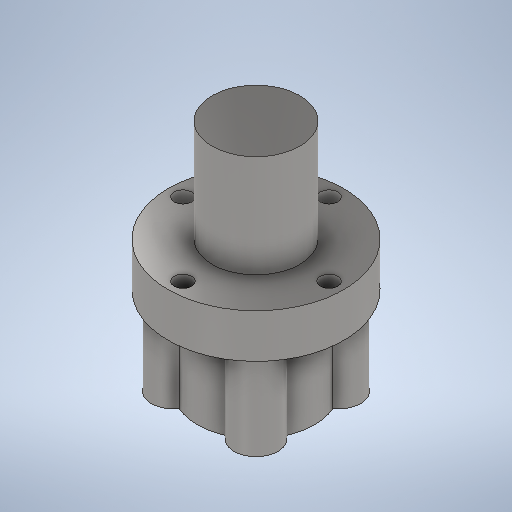
# Autodesk Inventor part: Крепление Барабана2
Saved by Autodesk Inventor 2025.1 (Build 291241000, 241)
## iProperties
Created: 2025-03-01
Part Number: Крепление Барабана2
Material: Сталь, литейная
Document SubType Name: Modeling
Designer: Timofey
Density: 7.85 g/cm^3
Appearance: С умеренной полировкой
Mass: 2001.3 g
Surface Area: 306.52 cm^2
Volume: 254.942 cm^3
Author: Timofey
Autodesk Inventor part; units mm, degrees
ref_plane "YZ Plane" through (0, 0, 0) normal (1, 0, 0) x (0, 1, 0)
ref_plane "XZ Plane" through (0, 0, 0) normal (0, 1, 0) x (-1, 0, 0)
ref_plane "XY Plane" through (0, 0, 0) normal (0, 0, 1) x (1, 0, 0)
sketch "Эскиз1" plane through (0, 0, 0) normal (0, 1, 0) x (-1, 0, 0)
  circle A0 centre (0, 0) radius 30
  dimension "d0" = 60
  constraints: 1 centre point, 1 coincident
  measures "d0" diameter of A0
extrude "Выдавливание1" add sketch "Эскиз1" along normal blind 15
sketch "Эскиз3" plane through (0, 0, 0) normal (0, -1, 0) x (1, 0, 0)
  circle A0 centre (0, 0) radius 20
  line L0 (0, 0) -> (30, 0) construction
  line L1 (0, 0) -> (30, 0) construction
  line L2 (0, 0) -> (30, 0) construction
  line L3 (0, 0) -> (30, 0) construction
  line L4 (0, 0) -> (14.1421, 14.1421)
  line L5 (0, 0) -> (20, 0) construction
  line L6 (0, 0) -> (14.1421, -14.1421)
  line L7 (0, 0) -> (-14.1421, 14.1421)
  line L8 (0, 0) -> (20, 0) construction
  line L9 (0, 0) -> (-14.1421, -14.1421)
  line L10 (0, 0) -> (20, 0) construction
  circle A1 centre (14.1421, 14.1421) radius 7.5
  circle A2 centre (14.1421, -14.1421) radius 7.5
  circle A3 centre (-14.1421, -14.1421) radius 7.5
  circle A4 centre (-14.1421, 14.1421) radius 7.5
  point P0 (-8.7707, -17.9743)
  point P1 (-16.2945, -11.5969)
  point P2 (-8.7707, 17.9743)
  point P3 (-16.2945, 11.5969)
  point P4 (11.5969, -16.2945)
  point P5 (17.9743, -8.7707)
  point P6 (17.995, 8.7282)
  point P7 (11.5862, 16.3021)
  point P8 (18.357, 7.9385)
  point P9 (7.9385, 18.357)
  point P10 (-7.9385, 18.357)
  point P11 (-18.357, 7.9385)
  point P12 (-18.357, -7.9385)
  point P13 (-7.9385, -18.357)
  point P14 (7.9385, -18.357)
  point P15 (18.357, -7.9385)
  dimension "d26" = 40
  dimension "d62" = 20
  dimension "d63" = 45
  dimension "d64" = 20
  dimension "d65" = 20
  dimension "d66" = 135
  dimension "d67" = 20
  dimension "d68" = 135
  dimension "d69" = 15
  dimension "d70" = 15
  dimension "d71" = 15
  dimension "d72" = 15
  constraints: 22 end point, 7 horizontal, 4 centre point, 3 coincident, 3 equal length, 2 point on line, 1 collinear, 1 perpendicular, 12 other
  measures "d62" distance of L0.start L4.end
  measures "d63" angle of L5 L4
  measures "d64" distance of L0.start L6.end
  measures "d65" distance of L0.start L7.end
  measures "d66" angle of L8 L7
  measures "d67" distance of L0.start L9.end
  measures "d68" angle of L9 L10
  measures "d69" diameter of A1
  measures "d70" diameter of A2
  measures "d71" diameter of A3
  measures "d72" diameter of A4
sketch "Эскиз4" plane through (0, 15, 0) normal (0, 1, 0) x (1, 0, 0)
  circle A0 centre (0, 0) radius 15
  dimension "d41" = 30
  constraints: 1 centre point, 1 coincident
  measures "d41" diameter of A0
extrude "Выдавливание3" add sketch "Эскиз4" along normal blind 35
sketch "Эскиз5" plane through (0, 15, 0) normal (0, 1, 0) x (1, 0, 0)
  line L0 (0, 0) -> (0, -25)
  arc A0 (20, 0) -> (20, 0) centre (0, 0) ccw projected
  line L1 (0, 0) -> (25, 0)
  line L2 (0, 0) -> (0, 25)
  line L3 (0, 0) -> (-25, 0)
  dimension "d44" = 25
  dimension "d45" = 25
  dimension "d46" = 25
  dimension "d47" = 25
  constraints: 8 end point, 2 horizontal, 2 vertical
  measures "d44" distance of L0.start L0.end
  measures "d45" distance of L1.start L1.end
  measures "d46" distance of L1.start L2.end
  measures "d47" distance of L1.start L3.end
hole "Отверстие3" at (0, 15, 25) at (-25, 15, 0) at (0, 15, -25) at (25, 15, 0) direction (0, -1, 0) diameter 6 end through all
extrude "Выдавливание4" add sketch "Эскиз3" along normal blind 30
